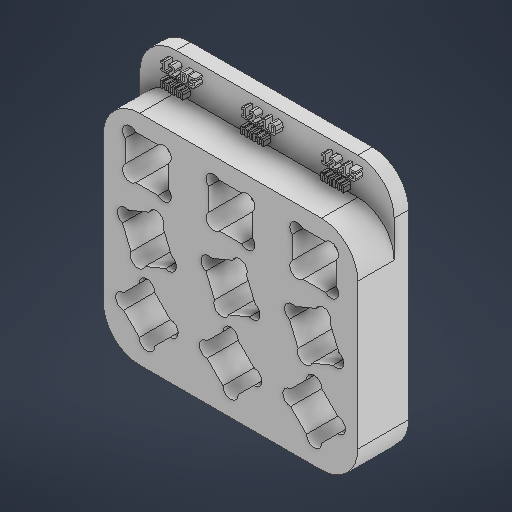
# Autodesk Inventor part: magnet_checker
Saved by Autodesk Inventor 2026.1 (Build 301233020, 233B)
## iProperties
Created: 2025-11-17
Part Number: magnet_checker
Material: Generic
Document SubType Name: Modeling
Designer: Carla Fernandez
Density: 1 g/cm^3
Appearance: Default
Author: Carla Fernandez
Autodesk Inventor part; units mm, degrees
ref_plane "YZ Plane" through (0, 0, 0) normal (1, 0, 0) x (0, 1, 0)
ref_plane "XZ Plane" through (0, 0, 0) normal (0, 1, 0) x (-1, 0, 0)
ref_plane "XY Plane" through (0, 0, 0) normal (0, 0, 1) x (1, 0, 0)
sketch "Sketch1" plane through (0, 0, 0) normal (0, 0, 1) x (1, 0, 0)
  line L0 (-35, 35) -> (35, 35)
  line L1 (35, 35) -> (35, -35)
  line L2 (35, -35) -> (-35, -35)
  line L3 (-35, -35) -> (-35, 35)
  point P0 (0, 0)
  point P1 (0, 35)
  point P2 (35, 0)
  dimension "d0" = 70
  dimension "d1" = 70
  constraints: 8 end point, 2 midpoint, 2 parallel, 1 horizontal, 1 horizontal alignment, 1 perpendicular, 1 vertical alignment
  measures "d0" distance of L2.end L0.start
  measures "d1" distance of L0.start L0.end
extrude "Extrusion1" add sketch "Sketch1" along normal blind 14
sketch "Sketch2" plane through (0, 0, 14) normal (0, 0, 1) x (1, 0, 0)
  line L0 (-29.025, 20) -> (-16.975, 20)
  line L1 (-16.975, 20) -> (-16.975, 7.95)
  line L2 (-16.975, 7.95) -> (-29.025, 7.95)
  line L3 (-29.025, 7.95) -> (-29.025, 20)
  line L4 (-35, 35) -> (-35, -35) projected
  line L5 (35, 35) -> (-35, 35) projected
  line L6 (-30.872, -0.7643) -> (-19.7393, 3.847)
  line L7 (-19.7393, 3.847) -> (-15.128, -7.2857)
  line L8 (-15.128, -7.2857) -> (-26.2607, -11.897)
  line L9 (-26.2607, -11.897) -> (-30.872, -0.7643)
  line L10 (-31.5206, -22.025) -> (-23, -13.5044)
  line L11 (-23, -13.5044) -> (-14.4794, -22.025)
  line L12 (-14.4794, -22.025) -> (-23, -30.5456)
  line L13 (-23, -30.5456) -> (-31.5206, -22.025)
  line L14 (-23, -30.5456) -> (-23, -13.5044) construction
  line L15 (-14.4794, -22.025) -> (-31.5206, -22.025) construction
  line L16 (-16.975, 20) -> (-29.025, 7.95) construction
  line L17 (-29.025, 20) -> (-16.975, 7.95) construction
  line L18 (-19.7393, 3.847) -> (-26.2607, -11.897) construction
  line L19 (-15.128, -7.2857) -> (-30.872, -0.7643) construction
  line L20 (-6.05, 20.025) -> (6.05, 20.025)
  line L21 (6.05, 20.025) -> (6.05, 7.925)
  line L22 (6.05, 7.925) -> (-6.05, 7.925)
  line L23 (-6.05, 7.925) -> (-6.05, 20.025)
  line L24 (-7.9047, -0.7508) -> (3.2742, 3.8797)
  line L25 (3.2742, 3.8797) -> (7.9047, -7.2992)
  line L26 (7.9047, -7.2992) -> (-3.2742, -11.9297)
  line L27 (-3.2742, -11.9297) -> (-7.9047, -0.7508)
  line L28 (-8.556, -22.025) -> (0, -13.469)
  line L29 (0, -13.469) -> (8.556, -22.025)
  line L30 (8.556, -22.025) -> (0, -30.581)
  line L31 (0, -30.581) -> (-8.556, -22.025)
  line L32 (0, -30.581) -> (0, -13.469) construction
  line L33 (8.556, -22.025) -> (-8.556, -22.025) construction
  line L34 (6.05, 20.025) -> (-6.05, 7.925) construction
  line L35 (-6.05, 20.025) -> (6.05, 7.925) construction
  line L36 (3.2742, 3.8797) -> (-3.2742, -11.9297) construction
  line L37 (7.9047, -7.2992) -> (-7.9047, -0.7508) construction
  line L38 (16.925, 20.05) -> (29.075, 20.05)
  line L39 (29.075, 20.05) -> (29.075, 7.9)
  line L40 (29.075, 7.9) -> (16.925, 7.9)
  line L41 (16.925, 7.9) -> (16.925, 20.05)
  line L42 (15.0626, -0.7372) -> (26.2878, 3.9124)
  line L43 (26.2878, 3.9124) -> (30.9374, -7.3128)
  line L44 (30.9374, -7.3128) -> (19.7122, -11.9624)
  line L45 (19.7122, -11.9624) -> (15.0626, -0.7372)
  line L46 (14.4087, -22.025) -> (23, -13.4337)
  line L47 (23, -13.4337) -> (31.5913, -22.025)
  line L48 (31.5913, -22.025) -> (23, -30.6163)
  line L49 (23, -30.6163) -> (14.4087, -22.025)
  line L50 (23, -30.6163) -> (23, -13.4337) construction
  line L51 (31.5913, -22.025) -> (14.4087, -22.025) construction
  line L52 (29.075, 20.05) -> (16.925, 7.9) construction
  line L53 (16.925, 20.05) -> (29.075, 7.9) construction
  line L54 (26.2878, 3.9124) -> (19.7122, -11.9624) construction
  line L55 (30.9374, -7.3128) -> (15.0626, -0.7372) construction
  line L56 (35, -35) -> (35, 35) construction
  point P0 (0, 0)
  point P1 (-23, 13.975)
  point P2 (-23, -22.025)
  point P3 (-23, 13.975)
  point P4 (-23, -4.025)
  point P5 (-23, -22.025)
  point P6 (0, 13.975)
  point P7 (0, -22.025)
  point P8 (0, 13.975)
  point P9 (0, -4.025)
  point P10 (0, -22.025)
  point P11 (23, 13.975)
  point P12 (23, -22.025)
  point P13 (23, 13.975)
  point P14 (23, -4.025)
  point P15 (23, -22.025)
  dimension "d4" = 12.05
  dimension "d6" = 15
  dimension "d9" = 18
  dimension "d10" = 18
  dimension "d11" = 22.5
  dimension "d12" = 12.1
  dimension "d15" = 18
  dimension "d16" = 18
  dimension "d17" = 22.5
  dimension "d18" = 12.15
  dimension "d21" = 18
  dimension "d22" = 18
  dimension "d23" = 22.5
  dimension "d24" = 12
  dimension "d25" = 12
  constraints: 108 end point, 18 midpoint, 18 parallel, 15 equal length, 15 perpendicular, 7 vertical alignment, 3 horizontal, 3 vertical, 2 horizontal alignment
  measures "d4" distance of L2.end L0.start
  measures "d6" distance between parallel lines of L0 L5
  measures "d9" distance of point (-23, -4.025) point (-23, 13.975)
  measures "d10" distance of point (-23, -22.025) point (-23, -4.025)
  measures "d11" angle of L2 L6
  measures "d12" distance of L23.start L20.start
  measures "d15" distance of point (0, -4.025) point (0, 13.975)
  measures "d16" distance of point (0, -22.025) point (0, -4.025)
  measures "d17" angle of L22 L24
  measures "d18" distance of L41.start L38.start
  measures "d21" distance of point (23, -4.025) point (23, 13.975)
  measures "d22" distance of point (23, -22.025) point (23, -4.025)
  measures "d23" angle of L40 L42
  measures "d24" distance from line of L56 point (23, 13.975)
  measures "d25" distance from line of L4 point (-23, 13.975)
extrude "Extrusion2" cut sketch "Sketch2" against normal blind 12
sketch "Sketch3" plane through (0, 0, 14) normal (0, 0, 1) x (1, 0, 0)
  circle A0 centre (-27.611, 18.586) radius 2.1
  circle A1 centre (-18.389, 18.586) radius 2.1
  circle A2 centre (-27.611, 9.364) radius 2.1
  circle A3 centre (-18.389, 9.364) radius 2.1
  line L0 (-29.025, 20) -> (-16.975, 7.95) construction
  line L1 (-29.025, 7.95) -> (-29.025, 20) construction
  line L2 (-29.025, 20) -> (-16.975, 20) construction
  line L3 (-16.975, 7.95) -> (-29.025, 7.95) construction
  line L4 (-16.975, 20) -> (-29.025, 7.95) construction
  line L5 (-30.872, -0.7643) -> (-19.7393, 3.847) construction
  line L6 (-15.128, -7.2857) -> (-26.2607, -11.897) construction
  line L7 (-19.7393, 3.847) -> (-26.2607, -11.897) construction
  line L8 (-26.2607, -11.897) -> (-30.872, -0.7643) construction
  line L9 (-15.128, -7.2857) -> (-30.872, -0.7643) construction
  line L10 (-31.5206, -22.025) -> (-23, -13.5044) construction
  line L11 (-23, -30.5456) -> (-31.5206, -22.025) construction
  line L12 (-23, -13.5044) -> (-23, -30.5456) construction
  line L13 (-14.4794, -22.025) -> (-23, -30.5456) construction
  line L14 (-31.5206, -22.025) -> (-14.4794, -22.025) construction
  circle A4 centre (-29.0246, -1.5295) radius 2.1
  circle A5 centre (-20.5045, 1.9996) radius 2.1
  circle A6 centre (-16.9754, -6.5205) radius 2.1
  circle A7 centre (-25.4955, -10.0496) radius 2.1
  line L15 (-19.7393, 3.847) -> (-15.128, -7.2857) projected
  circle A8 centre (-23, -15.5041) radius 2.1
  circle A9 centre (-16.4791, -22.025) radius 2.1
  circle A10 centre (-23, -28.5459) radius 2.1
  circle A11 centre (-29.5209, -22.025) radius 2.1
  line L16 (-23, -13.5044) -> (-14.4794, -22.025) projected
  circle A12 centre (-4.611, 18.586) radius 2.1
  circle A13 centre (-4.611, 9.364) radius 2.1
  circle A14 centre (4.611, 9.364) radius 2.1
  line L17 (-6.025, 20) -> (6.025, 7.95) construction
  line L18 (6.025, 20) -> (-6.025, 7.95) construction
  circle A15 centre (4.611, 18.586) radius 2.1
  line L19 (-8.5206, -22.025) -> (8.5206, -22.025) construction
  circle A16 centre (-6.5209, -22.025) radius 2.1
  circle A17 centre (6.5209, -22.025) radius 2.1
  circle A18 centre (0, -28.5459) radius 2.1
  line L20 (0, -13.5044) -> (0, -30.5456) construction
  circle A19 centre (2.4955, 1.9996) radius 2.1
  line L21 (7.872, -7.2857) -> (-7.872, -0.7643) construction
  circle A20 centre (6.0246, -6.5205) radius 2.1
  line L22 (3.2607, 3.847) -> (-3.2607, -11.897) construction
  circle A21 centre (-2.4955, -10.0496) radius 2.1
  circle A22 centre (0, -15.5041) radius 2.1
  circle A23 centre (-6.0246, -1.5295) radius 2.1
  circle A24 centre (18.389, 18.586) radius 2.1
  circle A25 centre (18.389, 9.364) radius 2.1
  circle A26 centre (27.611, 9.364) radius 2.1
  line L23 (16.975, 20) -> (29.025, 7.95) construction
  line L24 (29.025, 20) -> (16.975, 7.95) construction
  circle A27 centre (27.611, 18.586) radius 2.1
  line L25 (14.4794, -22.025) -> (31.5206, -22.025) construction
  circle A28 centre (16.4791, -22.025) radius 2.1
  circle A29 centre (29.5209, -22.025) radius 2.1
  circle A30 centre (23, -28.5459) radius 2.1
  line L26 (23, -13.5044) -> (23, -30.5456) construction
  circle A31 centre (25.4955, 1.9996) radius 2.1
  line L27 (30.872, -7.2857) -> (15.128, -0.7643) construction
  circle A32 centre (29.0246, -6.5205) radius 2.1
  line L28 (26.2607, 3.847) -> (19.7393, -11.897) construction
  circle A33 centre (20.5045, -10.0496) radius 2.1
  circle A34 centre (23, -15.5041) radius 2.1
  circle A35 centre (16.9754, -1.5295) radius 2.1
  point P0 (0, 0)
  dimension "d28" = 4.2
  dimension "d29" = 1.414
  dimension "d32" = 1.414
  dimension "d33" = 1.414
  dimension "d34" = 1.414
  dimension "d35" = 1.414
  dimension "d36" = 1.414
  dimension "d37" = 1.414
  dimension "d38" = 1.414
  dimension "d39" = 1.414
  dimension "d42" = 23
  constraints: 36 centre point, 36 end point, 33 point on line, 11 equal radius, 3 coincident, 2 horizontal, 2 horizontal alignment, 2 vertical alignment, 1 vertical, 86 other
  measures "d28" diameter of A0
  measures "d29" distance from line of A0.centre L1
  measures "d32" distance from line of L8 A4.centre
  measures "d33" distance from line of L15 A5.centre
  measures "d34" distance from line of L15 A6.centre
  measures "d35" distance from line of L6 A7.centre
  measures "d36" distance from line of L16 A8.centre
  measures "d37" distance from line of L13 A9.centre
  measures "d38" distance from line of A11.centre L10
  measures "d39" distance from line of L13 A10.centre
  measures "d42" distance of A0.centre A12.centre
extrude "Extrusion3" cut sketch "Sketch3" against normal blind 12
sketch "Sketch4" plane through (0, 0, 14) normal (0, 0, 1) x (1, 0, 0)
  circle A0 centre (-23, 13.975) radius 2
  line L0 (-29.025, 10.9166) -> (-29.025, 17.0334) projected
  line L1 (-26.0584, 20) -> (-19.9416, 20) projected
  circle A1 centre (-23, -4.025) radius 2
  circle A2 centre (-23, -22.025) radius 2
  circle A3 centre (0, 13.975) radius 2
  circle A4 centre (0, -4.025) radius 2
  circle A5 centre (0, -22.025) radius 2
  circle A6 centre (23, 13.975) radius 2
  circle A7 centre (23, -4.025) radius 2
  circle A8 centre (23, -22.025) radius 2
  point P0 (0, 0)
  point P1 (-29.025, 13.975)
  point P2 (-23, 20)
  dimension "d49" = 4
  dimension "d52" = 18
  dimension "d55" = 23
  constraints: 9 centre point, 2 midpoint, 1 horizontal, 1 horizontal alignment, 1 vertical, 1 vertical alignment, 16 other
  measures "d49" diameter of A0
  measures "d52" distance of A0.centre A1.centre
  measures "d55" distance of A0.centre A3.centre
extrude "Extrusion4" cut sketch "Sketch4" against normal through all
sketch "Sketch6" plane through (0, 0, 14) normal (0, 0, 1) x (1, 0, 0)
  line L0 (35, -35) -> (35, 35) projected
  line L1 (-35, 35) -> (35, 35)
  line L2 (35, 35) -> (35, 25)
  line L3 (35, 25) -> (-35, 25)
  line L4 (-35, 25) -> (-35, 35)
  point P0 (0, 0)
  dimension "d60" = 10
  constraints: 8 end point, 2 parallel, 1 horizontal, 1 perpendicular, 1 point on line
  measures "d60" distance between parallel lines of L3 L1
extrude "Extrusion5" cut sketch "Sketch6" against normal blind 10
sketch "Sketch5" plane through (0, 0, 4) normal (0, 0, 1) x (1, 0, 0)
  line L0 (-27.5814, 32.7858) -> (-13.7775, 32.7858) construction
  line L1 (-13.7775, 32.7858) -> (-13.7775, 28.2053) construction
  line L2 (-13.7775, 28.2053) -> (-27.5814, 28.2053) construction
  line L3 (-27.5814, 28.2053) -> (-27.5814, 32.7858) construction
  line L4 (-5.411, 32.7858) -> (5.411, 32.7858) construction
  line L5 (5.411, 32.7858) -> (5.411, 28.2053) construction
  line L6 (5.411, 28.2053) -> (-5.411, 28.2053) construction
  line L7 (-5.411, 28.2053) -> (-5.411, 32.7858) construction
  line L8 (16.6095, 32.7858) -> (30.4134, 32.7858) construction
  line L9 (30.4134, 32.7858) -> (30.4134, 28.2053) construction
  line L10 (30.4134, 28.2053) -> (16.6095, 28.2053) construction
  line L11 (16.6095, 28.2053) -> (16.6095, 32.7858) construction
  line L12 (-25.5704, 30.1943) -> (-27.248, 30.1943)
  line L13 (-27.248, 30.1943) -> (-27.248, 30.6369)
  line L14 (-27.248, 30.6369) -> (-26.7128, 30.6369)
  line L15 (-26.7128, 30.6369) -> (-26.7128, 31.981)
  line L16 (-26.7128, 31.981) -> (-27.248, 31.981)
  line L17 (-27.248, 31.981) -> (-27.248, 32.3947)
  spline S0 degree 2 poles (-27.248, 32.3947) (-27.1306, 32.3947) (-26.898, 32.4256) (-26.8281, 32.4585) knots 0 0 0 1 2 2 2
  spline S1 degree 2 poles (-26.8281, 32.4585) (-26.7478, 32.4997) (-26.6572, 32.6376) (-26.649, 32.7405) knots 0 0 0 1 2 2 2
  line L18 (-26.649, 32.7405) -> (-26.0932, 32.7405)
  line L19 (-26.0932, 32.7405) -> (-26.0932, 30.6369)
  line L20 (-26.0932, 30.6369) -> (-25.5704, 30.6369)
  line L21 (-25.5704, 30.6369) -> (-25.5704, 30.1943)
  line L22 (-23.2321, 30.1943) -> (-25.0991, 30.1943)
  line L23 (-25.0991, 30.1943) -> (-25.0991, 30.608)
  spline S2 degree 2 poles (-25.0991, 30.608) (-24.8623, 30.7974) (-24.4836, 31.1309) (-24.3416, 31.2811) knots 0 0 0 1 2 2 2
  spline S3 degree 2 poles (-24.3416, 31.2811) (-24.1543, 31.4767) (-23.9875, 31.7751) (-23.9875, 31.9316) knots 0 0 0 1 2 2 2
  spline S4 degree 2 poles (-23.9875, 31.9316) (-23.9875, 32.1086) (-24.1996, 32.298) (-24.3889, 32.298) knots 0 0 0 1 2 2 2
  spline S5 degree 2 poles (-24.3889, 32.298) (-24.4857, 32.298) (-24.6586, 32.2506) (-24.7471, 32.2136) knots 0 0 0 1 2 2 2
  spline S6 degree 2 poles (-24.7471, 32.2136) (-24.8335, 32.1745) (-24.957, 32.0921) (-24.9879, 32.0715) knots 0 0 0 1 2 2 2
  line L24 (-24.9879, 32.0715) -> (-25.0373, 32.0715)
  line L25 (-25.0373, 32.0715) -> (-25.0373, 32.6252)
  spline S7 degree 2 poles (-25.0373, 32.6252) (-24.9303, 32.6767) (-24.4733, 32.7837) (-24.2613, 32.7837) knots 0 0 0 1 2 2 2
  spline S8 degree 2 poles (-24.2613, 32.7837) (-23.8085, 32.7837) (-23.3433, 32.3803) (-23.3433, 32.016) knots 0 0 0 1 2 2 2
  spline S9 degree 2 poles (-23.3433, 32.016) (-23.3433, 31.7916) (-23.5553, 31.3593) (-23.8002, 31.1123) knots 0 0 0 1 2 2 2
  spline S10 degree 2 poles (-23.8002, 31.1123) (-23.9546, 30.96) (-24.2448, 30.7233) (-24.3086, 30.6739) knots 0 0 0 1 2 2 2
  line L26 (-24.3086, 30.6739) -> (-23.2321, 30.6739)
  line L27 (-23.2321, 30.6739) -> (-23.2321, 30.1943)
  line L28 (-22.2853, 30.1943) -> (-22.8884, 30.1943)
  line L29 (-22.8884, 30.1943) -> (-22.8884, 30.8653)
  line L30 (-22.8884, 30.8653) -> (-22.2853, 30.8653)
  line L31 (-22.2853, 30.8653) -> (-22.2853, 30.1943)
  spline S11 degree 2 poles (-19.9491, 31.4643) (-19.9491, 31.135) (-20.054, 30.641) (-20.1714, 30.4743) knots 0 0 0 1 2 2 2
  spline S12 degree 2 poles (-20.1714, 30.4743) (-20.2866, 30.3096) (-20.6592, 30.1408) (-20.9268, 30.1408) knots 0 0 0 1 2 2 2
  spline S13 degree 2 poles (-20.9268, 30.1408) (-21.1964, 30.1408) (-21.5669, 30.3096) (-21.6843, 30.4784) knots 0 0 0 1 2 2 2
  spline S14 degree 2 poles (-21.6843, 30.4784) (-21.8016, 30.6451) (-21.9066, 31.135) (-21.9066, 31.4643) knots 0 0 0 1 2 2 2
  spline S15 degree 2 poles (-21.9066, 31.4643) (-21.9066, 31.8019) (-21.8016, 32.2794) (-21.6822, 32.4523) knots 0 0 0 1 2 2 2
  spline S16 degree 2 poles (-21.6822, 32.4523) (-21.5628, 32.6211) (-21.1861, 32.7858) (-20.9268, 32.7858) knots 0 0 0 1 2 2 2
  spline S17 degree 2 poles (-20.9268, 32.7858) (-20.653, 32.7858) (-20.2866, 32.6129) (-20.1693, 32.442) knots 0 0 0 1 2 2 2
  spline S18 degree 2 poles (-20.1693, 32.442) (-20.054, 32.2753) (-19.9491, 31.7834) (-19.9491, 31.4643) knots 0 0 0 1 2 2 2
  spline S19 degree 2 poles (-20.5892, 31.4643) (-20.5892, 31.9357) (-20.7436, 32.3165) (-20.9268, 32.3165) knots 0 0 0 1 2 2 2
  spline S20 degree 2 poles (-20.9268, 32.3165) (-21.11, 32.3165) (-21.2664, 31.9357) (-21.2664, 31.4623) knots 0 0 0 1 2 2 2
  spline S21 degree 2 poles (-21.2664, 31.4623) (-21.2664, 30.9971) (-21.11, 30.6101) (-20.9268, 30.6101) knots 0 0 0 1 2 2 2
  spline S22 degree 2 poles (-20.9268, 30.6101) (-20.7456, 30.6101) (-20.5892, 30.9971) (-20.5892, 31.4643) knots 0 0 0 1 2 2 2
  spline S23 degree 2 poles (-17.7487, 31.0547) (-17.7487, 30.855) (-17.8845, 30.5175) (-18.0183, 30.396) knots 0 0 0 1 2 2 2
  spline S24 degree 2 poles (-18.0183, 30.396) (-18.1521, 30.2746) (-18.5185, 30.1408) (-18.7861, 30.1408) knots 0 0 0 1 2 2 2
  spline S25 degree 2 poles (-18.7861, 30.1408) (-19.0702, 30.1429) (-19.4777, 30.2355) (-19.6115, 30.2952) knots 0 0 0 1 2 2 2
  line L32 (-19.6115, 30.2952) -> (-19.6115, 30.8489)
  line L33 (-19.6115, 30.8489) -> (-19.5539, 30.8489)
  spline S26 degree 2 poles (-19.5539, 30.8489) (-19.5045, 30.8221) (-19.3851, 30.7521) (-19.2883, 30.7151) knots 0 0 0 1 2 2 2
  spline S27 degree 2 poles (-19.2883, 30.7151) (-19.1978, 30.6801) (-19.0105, 30.6327) (-18.8973, 30.6327) knots 0 0 0 1 2 2 2
  spline S28 degree 2 poles (-18.8973, 30.6327) (-18.7985, 30.6327) (-18.5679, 30.6821) (-18.4979, 30.748) knots 0 0 0 1 2 2 2
  spline S29 degree 2 poles (-18.4979, 30.748) (-18.4465, 30.7995) (-18.3888, 30.925) (-18.3888, 31.03) knots 0 0 0 1 2 2 2
  spline S30 degree 2 poles (-18.3888, 31.03) (-18.3888, 31.1206) (-18.4629, 31.2482) (-18.5226, 31.2873) knots 0 0 0 1 2 2 2
  spline S31 degree 2 poles (-18.5226, 31.2873) (-18.6091, 31.3449) (-18.8561, 31.3779) (-18.9446, 31.3779) knots 0 0 0 1 2 2 2
  spline S32 degree 2 poles (-18.9446, 31.3779) (-19.0846, 31.3779) (-19.3501, 31.3326) (-19.4468, 31.3079) knots 0 0 0 1 2 2 2
  line L34 (-19.4468, 31.3079) -> (-19.5024, 31.3079)
  line L35 (-19.5024, 31.3079) -> (-19.5024, 32.7343)
  line L36 (-19.5024, 32.7343) -> (-17.8187, 32.7343)
  line L37 (-17.8187, 32.7343) -> (-17.8187, 32.2547)
  line L38 (-17.8187, 32.2547) -> (-18.8993, 32.2547)
  line L39 (-18.8993, 32.2547) -> (-18.8993, 31.8328)
  spline S33 degree 2 poles (-18.8993, 31.8328) (-18.8479, 31.8369) (-18.7058, 31.841) (-18.6667, 31.841) knots 0 0 0 1 2 2 2
  spline S34 degree 2 poles (-18.6667, 31.841) (-18.4835, 31.841) (-18.1748, 31.7669) (-18.0533, 31.6907) knots 0 0 0 1 2 2 2
  spline S35 degree 2 poles (-18.0533, 31.6907) (-17.9092, 31.5961) (-17.7487, 31.2811) (-17.7487, 31.0547) knots 0 0 0 1 2 2 2
  line L40 (-25.0661, 26.0123) -> (-25.0661, 26.9694)
  spline S36 degree 2 poles (-25.0661, 26.9694) (-25.0661, 27.1114) (-25.0764, 27.3049) (-25.1011, 27.3667) knots 0 0 0 1 2 2 2
  spline S37 degree 2 poles (-25.1011, 27.3667) (-25.1279, 27.4284) (-25.2349, 27.484) (-25.3316, 27.484) knots 0 0 0 1 2 2 2
  spline S38 degree 2 poles (-25.3316, 27.484) (-25.3996, 27.484) (-25.5313, 27.4243) (-25.6095, 27.3687) knots 0 0 0 1 2 2 2
  line L41 (-25.6095, 27.3687) -> (-25.6095, 26.0123)
  line L42 (-25.6095, 26.0123) -> (-26.2106, 26.0123)
  line L43 (-26.2106, 26.0123) -> (-26.2106, 26.9694)
  spline S39 degree 2 poles (-26.2106, 26.9694) (-26.2106, 27.1094) (-26.2229, 27.3049) (-26.2476, 27.3667) knots 0 0 0 1 2 2 2
  spline S40 degree 2 poles (-26.2476, 27.3667) (-26.2744, 27.4284) (-26.3814, 27.484) (-26.4781, 27.484) knots 0 0 0 1 2 2 2
  spline S41 degree 2 poles (-26.4781, 27.484) (-26.5502, 27.484) (-26.6922, 27.4161) (-26.7581, 27.3687) knots 0 0 0 1 2 2 2
  line L44 (-26.7581, 27.3687) -> (-26.7581, 26.0123)
  line L45 (-26.7581, 26.0123) -> (-27.355, 26.0123)
  line L46 (-27.355, 26.0123) -> (-27.355, 27.9286)
  line L47 (-27.355, 27.9286) -> (-26.7581, 27.9286)
  line L48 (-26.7581, 27.9286) -> (-26.7581, 27.7166)
  spline S42 degree 2 poles (-26.7581, 27.7166) (-26.6119, 27.8401) (-26.3505, 27.9801) (-26.1879, 27.9801) knots 0 0 0 1 2 2 2
  spline S43 degree 2 poles (-26.1879, 27.9801) (-26.013, 27.9801) (-25.7454, 27.8133) (-25.6754, 27.6466) knots 0 0 0 1 2 2 2
  spline S44 degree 2 poles (-25.6754, 27.6466) (-25.5045, 27.8072) (-25.1999, 27.9801) (-25.0435, 27.9801) knots 0 0 0 1 2 2 2
  spline S45 degree 2 poles (-25.0435, 27.9801) (-24.9097, 27.9801) (-24.6977, 27.8957) (-24.6256, 27.8092) knots 0 0 0 1 2 2 2
  spline S46 degree 2 poles (-24.6256, 27.8092) (-24.5454, 27.7166) (-24.4651, 27.4634) (-24.4651, 27.2596) knots 0 0 0 1 2 2 2
  line L49 (-24.4651, 27.2596) -> (-24.4651, 26.0123)
  line L50 (-24.4651, 26.0123) -> (-25.0661, 26.0123)
  line L51 (-21.7357, 26.0123) -> (-21.7357, 26.9694)
  spline S47 degree 2 poles (-21.7357, 26.9694) (-21.7357, 27.1114) (-21.746, 27.3049) (-21.7707, 27.3667) knots 0 0 0 1 2 2 2
  spline S48 degree 2 poles (-21.7707, 27.3667) (-21.7975, 27.4284) (-21.9045, 27.484) (-22.0012, 27.484) knots 0 0 0 1 2 2 2
  spline S49 degree 2 poles (-22.0012, 27.484) (-22.0692, 27.484) (-22.2009, 27.4243) (-22.2791, 27.3687) knots 0 0 0 1 2 2 2
  line L52 (-22.2791, 27.3687) -> (-22.2791, 26.0123)
  line L53 (-22.2791, 26.0123) -> (-22.8802, 26.0123)
  line L54 (-22.8802, 26.0123) -> (-22.8802, 26.9694)
  spline S50 degree 2 poles (-22.8802, 26.9694) (-22.8802, 27.1094) (-22.8925, 27.3049) (-22.9172, 27.3667) knots 0 0 0 1 2 2 2
  spline S51 degree 2 poles (-22.9172, 27.3667) (-22.944, 27.4284) (-23.051, 27.484) (-23.1477, 27.484) knots 0 0 0 1 2 2 2
  spline S52 degree 2 poles (-23.1477, 27.484) (-23.2198, 27.484) (-23.3618, 27.4161) (-23.4277, 27.3687) knots 0 0 0 1 2 2 2
  line L55 (-23.4277, 27.3687) -> (-23.4277, 26.0123)
  line L56 (-23.4277, 26.0123) -> (-24.0246, 26.0123)
  line L57 (-24.0246, 26.0123) -> (-24.0246, 27.9286)
  line L58 (-24.0246, 27.9286) -> (-23.4277, 27.9286)
  line L59 (-23.4277, 27.9286) -> (-23.4277, 27.7166)
  spline S53 degree 2 poles (-23.4277, 27.7166) (-23.2815, 27.8401) (-23.0201, 27.9801) (-22.8575, 27.9801) knots 0 0 0 1 2 2 2
  spline S54 degree 2 poles (-22.8575, 27.9801) (-22.6826, 27.9801) (-22.415, 27.8133) (-22.345, 27.6466) knots 0 0 0 1 2 2 2
  spline S55 degree 2 poles (-22.345, 27.6466) (-22.1741, 27.8072) (-21.8695, 27.9801) (-21.7131, 27.9801) knots 0 0 0 1 2 2 2
  spline S56 degree 2 poles (-21.7131, 27.9801) (-21.5793, 27.9801) (-21.3673, 27.8957) (-21.2952, 27.8092) knots 0 0 0 1 2 2 2
  spline S57 degree 2 poles (-21.2952, 27.8092) (-21.215, 27.7166) (-21.1347, 27.4634) (-21.1347, 27.2596) knots 0 0 0 1 2 2 2
  line L60 (-21.1347, 27.2596) -> (-21.1347, 26.0123)
  line L61 (-21.1347, 26.0123) -> (-21.7357, 26.0123)
  line L62 (-3.4, 30.1943) -> (-5.0776, 30.1943)
  line L63 (-5.0776, 30.1943) -> (-5.0776, 30.6369)
  line L64 (-5.0776, 30.6369) -> (-4.5424, 30.6369)
  line L65 (-4.5424, 30.6369) -> (-4.5424, 31.981)
  line L66 (-4.5424, 31.981) -> (-5.0776, 31.981)
  line L67 (-5.0776, 31.981) -> (-5.0776, 32.3947)
  spline S58 degree 2 poles (-5.0776, 32.3947) (-4.9602, 32.3947) (-4.7276, 32.4256) (-4.6577, 32.4585) knots 0 0 0 1 2 2 2
  spline S59 degree 2 poles (-4.6577, 32.4585) (-4.5774, 32.4997) (-4.4868, 32.6376) (-4.4786, 32.7405) knots 0 0 0 1 2 2 2
  line L68 (-4.4786, 32.7405) -> (-3.9228, 32.7405)
  line L69 (-3.9228, 32.7405) -> (-3.9228, 30.6369)
  line L70 (-3.9228, 30.6369) -> (-3.4, 30.6369)
  line L71 (-3.4, 30.6369) -> (-3.4, 30.1943)
  line L72 (-1.0617, 30.1943) -> (-2.9287, 30.1943)
  line L73 (-2.9287, 30.1943) -> (-2.9287, 30.608)
  spline S60 degree 2 poles (-2.9287, 30.608) (-2.6919, 30.7974) (-2.3132, 31.1309) (-2.1712, 31.2811) knots 0 0 0 1 2 2 2
  spline S61 degree 2 poles (-2.1712, 31.2811) (-1.9839, 31.4767) (-1.8171, 31.7751) (-1.8171, 31.9316) knots 0 0 0 1 2 2 2
  spline S62 degree 2 poles (-1.8171, 31.9316) (-1.8171, 32.1086) (-2.0292, 32.298) (-2.2185, 32.298) knots 0 0 0 1 2 2 2
  spline S63 degree 2 poles (-2.2185, 32.298) (-2.3153, 32.298) (-2.4882, 32.2506) (-2.5767, 32.2136) knots 0 0 0 1 2 2 2
  spline S64 degree 2 poles (-2.5767, 32.2136) (-2.6631, 32.1745) (-2.7866, 32.0921) (-2.8175, 32.0715) knots 0 0 0 1 2 2 2
  line L74 (-2.8175, 32.0715) -> (-2.8669, 32.0715)
  line L75 (-2.8669, 32.0715) -> (-2.8669, 32.6252)
  spline S65 degree 2 poles (-2.8669, 32.6252) (-2.7599, 32.6767) (-2.3029, 32.7837) (-2.0909, 32.7837) knots 0 0 0 1 2 2 2
  spline S66 degree 2 poles (-2.0909, 32.7837) (-1.6381, 32.7837) (-1.1729, 32.3803) (-1.1729, 32.016) knots 0 0 0 1 2 2 2
  spline S67 degree 2 poles (-1.1729, 32.016) (-1.1729, 31.7916) (-1.3849, 31.3593) (-1.6298, 31.1123) knots 0 0 0 1 2 2 2
  spline S68 degree 2 poles (-1.6298, 31.1123) (-1.7842, 30.96) (-2.0744, 30.7233) (-2.1382, 30.6739) knots 0 0 0 1 2 2 2
  line L76 (-2.1382, 30.6739) -> (-1.0617, 30.6739)
  line L77 (-1.0617, 30.6739) -> (-1.0617, 30.1943)
  line L78 (-0.1149, 30.1943) -> (-0.718, 30.1943)
  line L79 (-0.718, 30.1943) -> (-0.718, 30.8653)
  line L80 (-0.718, 30.8653) -> (-0.1149, 30.8653)
  line L81 (-0.1149, 30.8653) -> (-0.1149, 30.1943)
  line L82 (2.1411, 30.1943) -> (0.4635, 30.1943)
  line L83 (0.4635, 30.1943) -> (0.4635, 30.6369)
  line L84 (0.4635, 30.6369) -> (0.9987, 30.6369)
  line L85 (0.9987, 30.6369) -> (0.9987, 31.981)
  line L86 (0.9987, 31.981) -> (0.4635, 31.981)
  line L87 (0.4635, 31.981) -> (0.4635, 32.3947)
  spline S69 degree 2 poles (0.4635, 32.3947) (0.5808, 32.3947) (0.8134, 32.4256) (0.8834, 32.4585) knots 0 0 0 1 2 2 2
  spline S70 degree 2 poles (0.8834, 32.4585) (0.9637, 32.4997) (1.0543, 32.6376) (1.0625, 32.7405) knots 0 0 0 1 2 2 2
  line L88 (1.0625, 32.7405) -> (1.6182, 32.7405)
  line L89 (1.6182, 32.7405) -> (1.6182, 30.6369)
  line L90 (1.6182, 30.6369) -> (2.1411, 30.6369)
  line L91 (2.1411, 30.6369) -> (2.1411, 30.1943)
  spline S71 degree 2 poles (4.4464, 31.4643) (4.4464, 31.135) (4.3414, 30.641) (4.2241, 30.4743) knots 0 0 0 1 2 2 2
  spline S72 degree 2 poles (4.2241, 30.4743) (4.1088, 30.3096) (3.7363, 30.1408) (3.4687, 30.1408) knots 0 0 0 1 2 2 2
  spline S73 degree 2 poles (3.4687, 30.1408) (3.199, 30.1408) (2.8285, 30.3096) (2.7112, 30.4784) knots 0 0 0 1 2 2 2
  spline S74 degree 2 poles (2.7112, 30.4784) (2.5939, 30.6451) (2.4889, 31.135) (2.4889, 31.4643) knots 0 0 0 1 2 2 2
  spline S75 degree 2 poles (2.4889, 31.4643) (2.4889, 31.8019) (2.5939, 32.2794) (2.7133, 32.4523) knots 0 0 0 1 2 2 2
  spline S76 degree 2 poles (2.7133, 32.4523) (2.8327, 32.6211) (3.2093, 32.7858) (3.4687, 32.7858) knots 0 0 0 1 2 2 2
  spline S77 degree 2 poles (3.4687, 32.7858) (3.7425, 32.7858) (4.1088, 32.6129) (4.2262, 32.442) knots 0 0 0 1 2 2 2
  spline S78 degree 2 poles (4.2262, 32.442) (4.3414, 32.2753) (4.4464, 31.7834) (4.4464, 31.4643) knots 0 0 0 1 2 2 2
  spline S79 degree 2 poles (3.8063, 31.4643) (3.8063, 31.9357) (3.6519, 32.3165) (3.4687, 32.3165) knots 0 0 0 1 2 2 2
  spline S80 degree 2 poles (3.4687, 32.3165) (3.2855, 32.3165) (3.1291, 31.9357) (3.1291, 31.4623) knots 0 0 0 1 2 2 2
  spline S81 degree 2 poles (3.1291, 31.4623) (3.1291, 30.9971) (3.2855, 30.6101) (3.4687, 30.6101) knots 0 0 0 1 2 2 2
  spline S82 degree 2 poles (3.4687, 30.6101) (3.6498, 30.6101) (3.8063, 30.9971) (3.8063, 31.4643) knots 0 0 0 1 2 2 2
  line L92 (-2.8957, 26.0123) -> (-2.8957, 26.9694)
  spline S83 degree 2 poles (-2.8957, 26.9694) (-2.8957, 27.1114) (-2.906, 27.3049) (-2.9307, 27.3667) knots 0 0 0 1 2 2 2
  spline S84 degree 2 poles (-2.9307, 27.3667) (-2.9575, 27.4284) (-3.0645, 27.484) (-3.1612, 27.484) knots 0 0 0 1 2 2 2
  spline S85 degree 2 poles (-3.1612, 27.484) (-3.2292, 27.484) (-3.3609, 27.4243) (-3.4391, 27.3687) knots 0 0 0 1 2 2 2
  line L93 (-3.4391, 27.3687) -> (-3.4391, 26.0123)
  line L94 (-3.4391, 26.0123) -> (-4.0402, 26.0123)
  line L95 (-4.0402, 26.0123) -> (-4.0402, 26.9694)
  spline S86 degree 2 poles (-4.0402, 26.9694) (-4.0402, 27.1094) (-4.0525, 27.3049) (-4.0772, 27.3667) knots 0 0 0 1 2 2 2
  spline S87 degree 2 poles (-4.0772, 27.3667) (-4.104, 27.4284) (-4.211, 27.484) (-4.3077, 27.484) knots 0 0 0 1 2 2 2
  spline S88 degree 2 poles (-4.3077, 27.484) (-4.3798, 27.484) (-4.5218, 27.4161) (-4.5877, 27.3687) knots 0 0 0 1 2 2 2
  line L96 (-4.5877, 27.3687) -> (-4.5877, 26.0123)
  line L97 (-4.5877, 26.0123) -> (-5.1846, 26.0123)
  line L98 (-5.1846, 26.0123) -> (-5.1846, 27.9286)
  line L99 (-5.1846, 27.9286) -> (-4.5877, 27.9286)
  line L100 (-4.5877, 27.9286) -> (-4.5877, 27.7166)
  spline S89 degree 2 poles (-4.5877, 27.7166) (-4.4415, 27.8401) (-4.1801, 27.9801) (-4.0175, 27.9801) knots 0 0 0 1 2 2 2
  spline S90 degree 2 poles (-4.0175, 27.9801) (-3.8426, 27.9801) (-3.575, 27.8133) (-3.505, 27.6466) knots 0 0 0 1 2 2 2
  spline S91 degree 2 poles (-3.505, 27.6466) (-3.3341, 27.8072) (-3.0295, 27.9801) (-2.8731, 27.9801) knots 0 0 0 1 2 2 2
  spline S92 degree 2 poles (-2.8731, 27.9801) (-2.7393, 27.9801) (-2.5273, 27.8957) (-2.4552, 27.8092) knots 0 0 0 1 2 2 2
  spline S93 degree 2 poles (-2.4552, 27.8092) (-2.375, 27.7166) (-2.2947, 27.4634) (-2.2947, 27.2596) knots 0 0 0 1 2 2 2
  line L101 (-2.2947, 27.2596) -> (-2.2947, 26.0123)
  line L102 (-2.2947, 26.0123) -> (-2.8957, 26.0123)
  line L103 (0.4347, 26.0123) -> (0.4347, 26.9694)
  spline S94 degree 2 poles (0.4347, 26.9694) (0.4347, 27.1114) (0.4244, 27.3049) (0.3997, 27.3667) knots 0 0 0 1 2 2 2
  spline S95 degree 2 poles (0.3997, 27.3667) (0.3729, 27.4284) (0.2659, 27.484) (0.1692, 27.484) knots 0 0 0 1 2 2 2
  spline S96 degree 2 poles (0.1692, 27.484) (0.1012, 27.484) (-0.0305, 27.4243) (-0.1087, 27.3687) knots 0 0 0 1 2 2 2
  line L104 (-0.1087, 27.3687) -> (-0.1087, 26.0123)
  line L105 (-0.1087, 26.0123) -> (-0.7098, 26.0123)
  line L106 (-0.7098, 26.0123) -> (-0.7098, 26.9694)
  spline S97 degree 2 poles (-0.7098, 26.9694) (-0.7098, 27.1094) (-0.7221, 27.3049) (-0.7468, 27.3667) knots 0 0 0 1 2 2 2
  spline S98 degree 2 poles (-0.7468, 27.3667) (-0.7736, 27.4284) (-0.8806, 27.484) (-0.9773, 27.484) knots 0 0 0 1 2 2 2
  spline S99 degree 2 poles (-0.9773, 27.484) (-1.0494, 27.484) (-1.1914, 27.4161) (-1.2573, 27.3687) knots 0 0 0 1 2 2 2
  line L107 (-1.2573, 27.3687) -> (-1.2573, 26.0123)
  line L108 (-1.2573, 26.0123) -> (-1.8542, 26.0123)
  line L109 (-1.8542, 26.0123) -> (-1.8542, 27.9286)
  line L110 (-1.8542, 27.9286) -> (-1.2573, 27.9286)
  line L111 (-1.2573, 27.9286) -> (-1.2573, 27.7166)
  spline S100 degree 2 poles (-1.2573, 27.7166) (-1.1111, 27.8401) (-0.8497, 27.9801) (-0.6871, 27.9801) knots 0 0 0 1 2 2 2
  spline S101 degree 2 poles (-0.6871, 27.9801) (-0.5122, 27.9801) (-0.2446, 27.8133) (-0.1746, 27.6466) knots 0 0 0 1 2 2 2
  spline S102 degree 2 poles (-0.1746, 27.6466) (-0.0037, 27.8072) (0.3009, 27.9801) (0.4573, 27.9801) knots 0 0 0 1 2 2 2
  spline S103 degree 2 poles (0.4573, 27.9801) (0.5911, 27.9801) (0.8031, 27.8957) (0.8752, 27.8092) knots 0 0 0 1 2 2 2
  spline S104 degree 2 poles (0.8752, 27.8092) (0.9554, 27.7166) (1.0357, 27.4634) (1.0357, 27.2596) knots 0 0 0 1 2 2 2
  line L112 (1.0357, 27.2596) -> (1.0357, 26.0123)
  line L113 (1.0357, 26.0123) -> (0.4347, 26.0123)
  line L114 (18.6205, 30.1964) -> (16.9429, 30.1964)
  line L115 (16.9429, 30.1964) -> (16.9429, 30.6389)
  line L116 (16.9429, 30.6389) -> (17.4781, 30.6389)
  line L117 (17.4781, 30.6389) -> (17.4781, 31.983)
  line L118 (17.4781, 31.983) -> (16.9429, 31.983)
  line L119 (16.9429, 31.983) -> (16.9429, 32.3968)
  spline S105 degree 2 poles (16.9429, 32.3968) (17.0603, 32.3968) (17.2929, 32.4276) (17.3628, 32.4606) knots 0 0 0 1 2 2 2
  spline S106 degree 2 poles (17.3628, 32.4606) (17.4431, 32.5017) (17.5337, 32.6396) (17.5419, 32.7426) knots 0 0 0 1 2 2 2
  line L120 (17.5419, 32.7426) -> (18.0977, 32.7426)
  line L121 (18.0977, 32.7426) -> (18.0977, 30.6389)
  line L122 (18.0977, 30.6389) -> (18.6205, 30.6389)
  line L123 (18.6205, 30.6389) -> (18.6205, 30.1964)
  line L124 (20.9588, 30.1964) -> (19.0919, 30.1964)
  line L125 (19.0919, 30.1964) -> (19.0919, 30.6101)
  spline S107 degree 2 poles (19.0919, 30.6101) (19.3286, 30.7995) (19.7073, 31.1329) (19.8493, 31.2832) knots 0 0 0 1 2 2 2
  spline S108 degree 2 poles (19.8493, 31.2832) (20.0366, 31.4787) (20.2034, 31.7772) (20.2034, 31.9336) knots 0 0 0 1 2 2 2
  spline S109 degree 2 poles (20.2034, 31.9336) (20.2034, 32.1106) (19.9914, 32.3) (19.802, 32.3) knots 0 0 0 1 2 2 2
  spline S110 degree 2 poles (19.802, 32.3) (19.7052, 32.3) (19.5323, 32.2527) (19.4438, 32.2156) knots 0 0 0 1 2 2 2
  spline S111 degree 2 poles (19.4438, 32.2156) (19.3574, 32.1765) (19.2339, 32.0942) (19.203, 32.0736) knots 0 0 0 1 2 2 2
  line L126 (19.203, 32.0736) -> (19.1536, 32.0736)
  line L127 (19.1536, 32.0736) -> (19.1536, 32.6273)
  spline S112 degree 2 poles (19.1536, 32.6273) (19.2606, 32.6787) (19.7176, 32.7858) (19.9296, 32.7858) knots 0 0 0 1 2 2 2
  spline S113 degree 2 poles (19.9296, 32.7858) (20.3824, 32.7858) (20.8476, 32.3823) (20.8476, 32.018) knots 0 0 0 1 2 2 2
  spline S114 degree 2 poles (20.8476, 32.018) (20.8476, 31.7937) (20.6356, 31.3614) (20.3907, 31.1144) knots 0 0 0 1 2 2 2
  spline S115 degree 2 poles (20.3907, 31.1144) (20.2363, 30.9621) (19.9461, 30.7254) (19.8823, 30.676) knots 0 0 0 1 2 2 2
  line L128 (19.8823, 30.676) -> (20.9588, 30.676)
  line L129 (20.9588, 30.676) -> (20.9588, 30.1964)
  line L130 (21.9056, 30.1964) -> (21.3025, 30.1964)
  line L131 (21.3025, 30.1964) -> (21.3025, 30.8674)
  line L132 (21.3025, 30.8674) -> (21.9056, 30.8674)
  line L133 (21.9056, 30.8674) -> (21.9056, 30.1964)
  line L134 (24.1616, 30.1964) -> (22.484, 30.1964)
  line L135 (22.484, 30.1964) -> (22.484, 30.6389)
  line L136 (22.484, 30.6389) -> (23.0192, 30.6389)
  line L137 (23.0192, 30.6389) -> (23.0192, 31.983)
  line L138 (23.0192, 31.983) -> (22.484, 31.983)
  line L139 (22.484, 31.983) -> (22.484, 32.3968)
  spline S116 degree 2 poles (22.484, 32.3968) (22.6013, 32.3968) (22.8339, 32.4276) (22.9039, 32.4606) knots 0 0 0 1 2 2 2
  spline S117 degree 2 poles (22.9039, 32.4606) (22.9842, 32.5017) (23.0748, 32.6396) (23.083, 32.7426) knots 0 0 0 1 2 2 2
  line L140 (23.083, 32.7426) -> (23.6387, 32.7426)
  line L141 (23.6387, 32.7426) -> (23.6387, 30.6389)
  line L142 (23.6387, 30.6389) -> (24.1616, 30.6389)
  line L143 (24.1616, 30.6389) -> (24.1616, 30.1964)
  spline S118 degree 2 poles (26.4422, 31.0568) (26.4422, 30.8571) (26.3064, 30.5195) (26.1726, 30.3981) knots 0 0 0 1 2 2 2
  spline S119 degree 2 poles (26.1726, 30.3981) (26.0388, 30.2767) (25.6724, 30.1429) (25.4048, 30.1429) knots 0 0 0 1 2 2 2
  spline S120 degree 2 poles (25.4048, 30.1429) (25.1208, 30.1449) (24.7132, 30.2375) (24.5794, 30.2972) knots 0 0 0 1 2 2 2
  line L144 (24.5794, 30.2972) -> (24.5794, 30.8509)
  line L145 (24.5794, 30.8509) -> (24.637, 30.8509)
  spline S121 degree 2 poles (24.637, 30.8509) (24.6864, 30.8242) (24.8058, 30.7542) (24.9026, 30.7171) knots 0 0 0 1 2 2 2
  spline S122 degree 2 poles (24.9026, 30.7171) (24.9931, 30.6821) (25.1804, 30.6348) (25.2937, 30.6348) knots 0 0 0 1 2 2 2
  spline S123 degree 2 poles (25.2937, 30.6348) (25.3925, 30.6348) (25.623, 30.6842) (25.693, 30.7501) knots 0 0 0 1 2 2 2
  spline S124 degree 2 poles (25.693, 30.7501) (25.7444, 30.8015) (25.8021, 30.9271) (25.8021, 31.0321) knots 0 0 0 1 2 2 2
  spline S125 degree 2 poles (25.8021, 31.0321) (25.8021, 31.1226) (25.728, 31.2503) (25.6683, 31.2894) knots 0 0 0 1 2 2 2
  spline S126 degree 2 poles (25.6683, 31.2894) (25.5818, 31.347) (25.3348, 31.3799) (25.2463, 31.3799) knots 0 0 0 1 2 2 2
  spline S127 degree 2 poles (25.2463, 31.3799) (25.1063, 31.3799) (24.8408, 31.3346) (24.7441, 31.3099) knots 0 0 0 1 2 2 2
  line L146 (24.7441, 31.3099) -> (24.6885, 31.3099)
  line L147 (24.6885, 31.3099) -> (24.6885, 32.7364)
  line L148 (24.6885, 32.7364) -> (26.3722, 32.7364)
  line L149 (26.3722, 32.7364) -> (26.3722, 32.2568)
  line L150 (26.3722, 32.2568) -> (25.2916, 32.2568)
  line L151 (25.2916, 32.2568) -> (25.2916, 31.8348)
  spline S128 degree 2 poles (25.2916, 31.8348) (25.3431, 31.8389) (25.4851, 31.8431) (25.5242, 31.8431) knots 0 0 0 1 2 2 2
  spline S129 degree 2 poles (25.5242, 31.8431) (25.7074, 31.8431) (26.0161, 31.769) (26.1376, 31.6928) knots 0 0 0 1 2 2 2
  spline S130 degree 2 poles (26.1376, 31.6928) (26.2817, 31.5981) (26.4422, 31.2832) (26.4422, 31.0568) knots 0 0 0 1 2 2 2
  line L152 (19.1248, 26.0143) -> (19.1248, 26.9715)
  spline S131 degree 2 poles (19.1248, 26.9715) (19.1248, 27.1135) (19.1145, 27.307) (19.0898, 27.3687) knots 0 0 0 1 2 2 2
  spline S132 degree 2 poles (19.0898, 27.3687) (19.063, 27.4305) (18.956, 27.4861) (18.8593, 27.4861) knots 0 0 0 1 2 2 2
  spline S133 degree 2 poles (18.8593, 27.4861) (18.7913, 27.4861) (18.6596, 27.4264) (18.5814, 27.3708) knots 0 0 0 1 2 2 2
  line L153 (18.5814, 27.3708) -> (18.5814, 26.0143)
  line L154 (18.5814, 26.0143) -> (17.9803, 26.0143)
  line L155 (17.9803, 26.0143) -> (17.9803, 26.9715)
  spline S134 degree 2 poles (17.9803, 26.9715) (17.9803, 27.1114) (17.968, 27.307) (17.9433, 27.3687) knots 0 0 0 1 2 2 2
  spline S135 degree 2 poles (17.9433, 27.3687) (17.9165, 27.4305) (17.8095, 27.4861) (17.7128, 27.4861) knots 0 0 0 1 2 2 2
  spline S136 degree 2 poles (17.7128, 27.4861) (17.6407, 27.4861) (17.4987, 27.4181) (17.4328, 27.3708) knots 0 0 0 1 2 2 2
  line L156 (17.4328, 27.3708) -> (17.4328, 26.0143)
  line L157 (17.4328, 26.0143) -> (16.8359, 26.0143)
  line L158 (16.8359, 26.0143) -> (16.8359, 27.9307)
  line L159 (16.8359, 27.9307) -> (17.4328, 27.9307)
  line L160 (17.4328, 27.9307) -> (17.4328, 27.7186)
  spline S137 degree 2 poles (17.4328, 27.7186) (17.579, 27.8421) (17.8404, 27.9821) (18.003, 27.9821) knots 0 0 0 1 2 2 2
  spline S138 degree 2 poles (18.003, 27.9821) (18.1779, 27.9821) (18.4455, 27.8154) (18.5155, 27.6487) knots 0 0 0 1 2 2 2
  spline S139 degree 2 poles (18.5155, 27.6487) (18.6864, 27.8092) (18.991, 27.9821) (19.1474, 27.9821) knots 0 0 0 1 2 2 2
  spline S140 degree 2 poles (19.1474, 27.9821) (19.2812, 27.9821) (19.4932, 27.8977) (19.5653, 27.8113) knots 0 0 0 1 2 2 2
  spline S141 degree 2 poles (19.5653, 27.8113) (19.6455, 27.7186) (19.7258, 27.4655) (19.7258, 27.2617) knots 0 0 0 1 2 2 2
  line L161 (19.7258, 27.2617) -> (19.7258, 26.0143)
  line L162 (19.7258, 26.0143) -> (19.1248, 26.0143)
  line L163 (22.4552, 26.0143) -> (22.4552, 26.9715)
  spline S142 degree 2 poles (22.4552, 26.9715) (22.4552, 27.1135) (22.4449, 27.307) (22.4202, 27.3687) knots 0 0 0 1 2 2 2
  spline S143 degree 2 poles (22.4202, 27.3687) (22.3934, 27.4305) (22.2864, 27.4861) (22.1897, 27.4861) knots 0 0 0 1 2 2 2
  spline S144 degree 2 poles (22.1897, 27.4861) (22.1217, 27.4861) (21.99, 27.4264) (21.9118, 27.3708) knots 0 0 0 1 2 2 2
  line L164 (21.9118, 27.3708) -> (21.9118, 26.0143)
  line L165 (21.9118, 26.0143) -> (21.3108, 26.0143)
  line L166 (21.3108, 26.0143) -> (21.3108, 26.9715)
  spline S145 degree 2 poles (21.3108, 26.9715) (21.3108, 27.1114) (21.2984, 27.307) (21.2737, 27.3687) knots 0 0 0 1 2 2 2
  spline S146 degree 2 poles (21.2737, 27.3687) (21.2469, 27.4305) (21.1399, 27.4861) (21.0432, 27.4861) knots 0 0 0 1 2 2 2
  spline S147 degree 2 poles (21.0432, 27.4861) (20.9711, 27.4861) (20.8291, 27.4181) (20.7632, 27.3708) knots 0 0 0 1 2 2 2
  line L167 (20.7632, 27.3708) -> (20.7632, 26.0143)
  line L168 (20.7632, 26.0143) -> (20.1663, 26.0143)
  line L169 (20.1663, 26.0143) -> (20.1663, 27.9307)
  line L170 (20.1663, 27.9307) -> (20.7632, 27.9307)
  line L171 (20.7632, 27.9307) -> (20.7632, 27.7186)
  spline S148 degree 2 poles (20.7632, 27.7186) (20.9094, 27.8421) (21.1708, 27.9821) (21.3334, 27.9821) knots 0 0 0 1 2 2 2
  spline S149 degree 2 poles (21.3334, 27.9821) (21.5084, 27.9821) (21.7759, 27.8154) (21.8459, 27.6487) knots 0 0 0 1 2 2 2
  spline S150 degree 2 poles (21.8459, 27.6487) (22.0168, 27.8092) (22.3214, 27.9821) (22.4778, 27.9821) knots 0 0 0 1 2 2 2
  spline S151 degree 2 poles (22.4778, 27.9821) (22.6116, 27.9821) (22.8236, 27.8977) (22.8957, 27.8113) knots 0 0 0 1 2 2 2
  spline S152 degree 2 poles (22.8957, 27.8113) (22.976, 27.7186) (23.0562, 27.4655) (23.0562, 27.2617) knots 0 0 0 1 2 2 2
  line L172 (23.0562, 27.2617) -> (23.0562, 26.0143)
  line L173 (23.0562, 26.0143) -> (22.4552, 26.0143)
  point P0 (0, 0)
  point P1 (0, 32.7858)
  dimension "d0" = 70
  dimension "d1" = 70
  constraints: 2 horizontal alignment, 1 midpoint, 1 vertical alignment, 6 other
emboss "Emboss1" sketch "Sketch5" operation add depth 2 direction (0, 0, -1)
fillet "Fillet1" radius 10 6 edges at (35, 25, 9) (35, 35, 2) (-35, 35, 2) (-35, 25, 9) (-35, -35, 7) (35, -35, 7)
body "Solid1"
